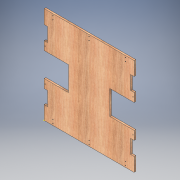
# Autodesk Inventor part: Belly Pan
Saved by Autodesk Inventor 2019 (Build 230136000, 136)
## iProperties
Created: 2018-11-11
Part Number: Belly Pan
Material: Wood (Birch)
Document SubType Name: Modeling
Designer: maste
Density: 0.55 g/cm^3
Appearance: Birch - Natural Polished
Author: maste
Autodesk Inventor part; units mm, degrees
ref_plane "YZ Plane" through (0, 0, 0) normal (1, 0, 0) x (0, 1, 0)
ref_plane "XZ Plane" through (0, 0, 0) normal (0, 1, 0) x (-1, 0, 0)
ref_plane "XY Plane" through (0, 0, 0) normal (0, 0, 1) x (1, 0, 0)
sketch "Sketch1" plane through (0, 0, 0) normal (0, 0, 1) x (1, 0, 0)
  line L0 (0, 0) -> (660.4, 0)
  line L1 (660.4, 711.2) -> (0, 711.2)
  line L2 (0, 0) -> (0, 50.8)
  line L3 (660.4, 711.2) -> (660.4, 660.4)
  line L4 (0, 50.8) -> (0, 101.6)
  line L5 (0, 101.6) -> (25.4, 101.6)
  line L6 (25.4, 101.6) -> (25.4, 177.8)
  line L7 (25.4, 177.8) -> (0, 177.8)
  line L8 (0, 177.8) -> (0, 266.7)
  line L9 (0, 266.7) -> (177.8, 266.7)
  line L10 (177.8, 266.7) -> (177.8, 355.6)
  line L11 (0, 609.6) -> (25.4, 609.6)
  line L12 (25.4, 609.6) -> (25.4, 533.4)
  line L13 (25.4, 533.4) -> (0, 533.4)
  line L14 (0, 444.5) -> (177.8, 444.5)
  line L15 (177.8, 444.5) -> (177.8, 355.6)
  line L16 (660.4, 101.6) -> (635, 101.6)
  line L17 (635, 101.6) -> (635, 177.8)
  line L18 (635, 177.8) -> (660.4, 177.8)
  line L19 (660.4, 609.6) -> (635, 609.6)
  line L20 (635, 609.6) -> (635, 533.4)
  line L21 (635, 533.4) -> (660.4, 533.4)
  line L22 (0, 711.2) -> (0, 609.6)
  line L23 (660.4, 609.6) -> (660.4, 711.2)
  line L24 (660.4, 444.5) -> (660.4, 533.4)
  line L25 (660.4, 0) -> (660.4, 101.6)
  line L26 (660.4, 177.8) -> (660.4, 266.7)
  line L27 (0, 101.6) -> (0, 0)
  line L28 (0, 533.4) -> (0, 444.5)
  line L29 (0, 266.7) -> (0, 177.8)
  line L30 (660.4, 444.5) -> (482.6, 444.5)
  line L31 (482.6, 444.5) -> (482.6, 266.7)
  line L32 (482.6, 266.7) -> (660.4, 266.7)
  dimension "d0" = 660.4
  dimension "d1" = 711.2
  dimension "d2" = 50.8
  dimension "d3" = 50.8
  dimension "d4" = 50.8
  dimension "d5" = 25.4
  dimension "d6" = 76.2
  dimension "d7" = 88.9
  dimension "d8" = 177.8
  dimension "d24" = 177.8
  constraints: 66 end point, 17 parallel, 9 perpendicular, 2 horizontal, 2 midpoint, 1 vertical
  measures "d0" distance of L1.end L1.start
  measures "d1" distance of L1.start L0.end
  measures "d2" distance of L0.start L2.end
  measures "d3" distance of L1.start L3.end
  measures "d4" distance of L2.end L4.end
  measures "d5" distance of L4.end L5.end
  measures "d6" distance of L5.end L6.end
  measures "d7" distance of L7.end L8.end
  measures "d8" distance of L8.end L9.end
  measures "d24" distance of L24.start L30.end
extrude "Extrusion1" add sketch "Sketch1" along normal blind 12.7
sketch "Sketch2" plane through (0, 0, 12.7) normal (0, 0, 1) x (1, 0, 0)
  line L0 (0, 0) -> (660.4, 0) projected
  line L1 (330.2, 0) -> (330.2, 711.2)
  line L2 (660.4, 711.2) -> (0, 711.2) projected
  line L3 (0, 355.6) -> (660.4, 355.6)
  line L4 (558.8, 444.5) -> (660.4, 444.5) projected
  line L5 (0, 234.95) -> (7.9375, 234.95)
  circle A0 centre (7.9375, 234.95) radius 2.54
  circle A1 centre (7.9375, 476.25) radius 2.54
  circle A2 centre (652.4625, 234.95) radius 2.54
  circle A3 centre (652.4625, 476.25) radius 2.54
  line L6 (0, 0) -> (63.5, 0)
  line L7 (63.5, 0) -> (63.5, 12.7)
  line L8 (63.5, 12.7) -> (63.5, 38.1)
  circle A4 centre (63.5, 12.7) radius 2.54
  circle A5 centre (63.5, 38.1) radius 2.54
  circle A6 centre (596.9, 12.7) radius 2.54
  circle A7 centre (596.9, 38.1) radius 2.54
  circle A8 centre (63.5, 698.5) radius 2.54
  circle A9 centre (63.5, 673.1) radius 2.54
  circle A10 centre (596.9, 673.1) radius 2.54
  circle A11 centre (596.9, 698.5) radius 2.54
  line L9 (330.2, 0) -> (330.2, 12.7)
  line L10 (330.2, 12.7) -> (330.2, 38.1)
  circle A12 centre (330.2, 12.7) radius 2.54
  circle A13 centre (330.2, 38.1) radius 2.54
  circle A14 centre (330.2, 698.5) radius 2.54
  circle A15 centre (330.2, 673.1) radius 2.54
  line L11 (177.8, 266.7) -> (0, 266.7) projected
  point P0 (0, 177.8)
  dimension "d11" = 7.9375
  dimension "d12" = 5.08
  dimension "d13" = 63.5
  dimension "d14" = 12.7
  dimension "d15" = 25.4
  dimension "d16" = 5.08
  dimension "d17" = 5.08
  dimension "d18" = 12.7
  dimension "d19" = 25.4
  dimension "d20" = 5.08
  dimension "d21" = 5.08
  dimension "d28" = 31.75
  constraints: 16 centre point, 16 end point, 11 symmetric about line, 5 coincident, 4 point on line, 2 midpoint, 1 horizontal, 1 parallel, 1 perpendicular, 11 other
  measures "d11" distance of L5.start L5.end
  measures "d12" diameter of A0
  measures "d13" distance of L0.start L6.end
  measures "d14" distance of L6.end L7.end
  measures "d15" distance of L7.end L8.end
  measures "d16" diameter of A4
  measures "d17" diameter of A5
  measures "d18" distance of L1.start L9.end
  measures "d19" distance of L9.end L10.end
  measures "d20" diameter of A12
  measures "d21" diameter of A13
  measures "d28" distance between parallel lines of L11 L5
extrude "Extrusion2" cut sketch "Sketch2" against normal blind 25.4
sketch "Sketch3" plane through (0, 0, 12.7) normal (0, 0, 1) x (1, 0, 0)
  line L0 (25.4, 609.6) -> (25.4, 533.4) projected
  line L1 (25.4, 533.4) -> (25.4, 508)
  line L2 (25.4, 508) -> (0, 508)
  line L3 (0, 533.4) -> (0, 444.5) projected
  line L4 (0, 508) -> (0, 533.4)
  line L5 (25.4, 533.4) -> (0, 533.4) projected
  line L6 (0, 533.4) -> (25.4, 533.4)
  line L7 (660.4, 711.2) -> (0, 711.2) projected
  line L8 (330.2, 711.2) -> (330.2, 0)
  line L9 (0, 0) -> (660.4, 0) projected
  line L10 (0, 355.6) -> (660.4, 355.6)
  line L11 (635, 533.4) -> (635, 508)
  line L12 (635, 508) -> (660.4, 508)
  line L13 (660.4, 533.4) -> (660.4, 444.5)
  line L14 (635, 533.4) -> (660.4, 533.4)
  line L15 (25.4, 101.6) -> (25.4, 177.8)
  line L16 (25.4, 177.8) -> (25.4, 203.2)
  line L17 (25.4, 203.2) -> (0, 203.2)
  line L18 (0, 177.8) -> (0, 266.7)
  line L19 (0, 203.2) -> (0, 177.8)
  line L20 (25.4, 177.8) -> (0, 177.8)
  line L21 (0, 177.8) -> (25.4, 177.8)
  line L22 (635, 177.8) -> (635, 203.2)
  line L23 (635, 203.2) -> (660.4, 203.2)
  line L24 (660.4, 177.8) -> (660.4, 266.7)
  line L25 (635, 177.8) -> (660.4, 177.8)
  dimension "d25" = 25.4
  constraints: 42 end point, 17 symmetric about line, 4 point on line, 2 midpoint, 2 perpendicular, 2 vertical, 1 horizontal
  measures "d25" distance of L0.end L1.end
extrude "Extrusion3" cut sketch "Sketch3" against normal blind 25.4
sketch "Sketch4" plane through (0, 0, 12.7) normal (0, 0, 1) x (1, 0, 0)
  point P0 (0, 0)
body "Solid1"
